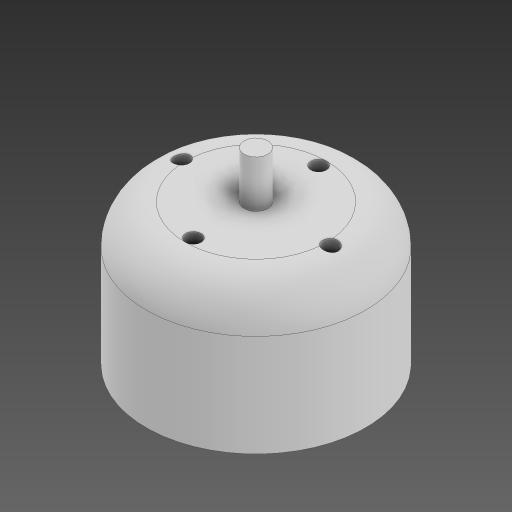
# Autodesk Inventor part: motor_c2822
Saved by Autodesk Inventor 2023 (Build 270158000, 158)
## iProperties
Created: 2025-05-25
Part Number: motor_c2822
Material: Типовые
Document SubType Name: Modeling
Designer: daa
Density: 1 g/cm^3
Appearance: По умолчанию
Author: daa
Autodesk Inventor part; units mm, degrees
ref_plane "YZ Plane" through (0, 0, 0) normal (1, 0, 0) x (0, 1, 0)
ref_plane "XZ Plane" through (0, 0, 0) normal (0, 1, 0) x (-1, 0, 0)
ref_plane "XY Plane" through (0, 0, 0) normal (0, 0, 1) x (1, 0, 0)
sketch "Эскиз1" plane through (0, 0, 0) normal (0, 1, 0) x (-1, 0, 0)
  circle A0 centre (0, 0) radius 14
  dimension "d0" = 28
  constraints: 1 centre point, 1 coincident
  measures "d0" diameter of A0
extrude "Выдавливание1" add sketch "Эскиз1" along normal blind 18
sketch "Эскиз2" plane through (0, 18, 0) normal (0, 1, 0) x (1, 0, 0)
  circle A0 centre (0, 0) radius 1.5
  dimension "d3" = 3
  constraints: 1 centre point, 1 coincident
  measures "d3" diameter of A0
extrude "Выдавливание2" add sketch "Эскиз2" along normal blind 6
sketch "Эскиз3" plane through (0, 18, 0) normal (0, 1, 0) x (1, 0, 0)
  circle A0 centre (0, 8) radius 1
  circle A1 centre (0, -8) radius 1
  circle A2 centre (-9.5, 0) radius 1
  circle A3 centre (9.5, 0) radius 1
  point P0 (0, 0)
  dimension "d6" = 2
  dimension "d7" = 2
  dimension "d8" = 2
  dimension "d9" = 2
  dimension "d10" = 8
  dimension "d11" = 8
  dimension "d12" = 9.5
  dimension "d13" = 9.5
  constraints: 4 centre point
  measures "d6" diameter of A0
  measures "d7" diameter of A1
  measures "d8" diameter of A2
  measures "d9" diameter of A3
  measures "d10" distance of A0.centre point (0, 0)
  measures "d11" distance of A1.centre point (0, 0)
  measures "d12" distance of A3.centre point (0, 0)
  measures "d13" distance of point (0, 0) A2.centre
extrude "Выдавливание3" cut sketch "Эскиз3" against normal blind 5
fillet "Сопряжение1" radius 5 1 edges at (14, 18, 0)
